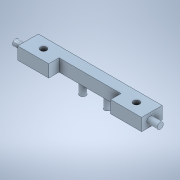
# Autodesk Inventor part: Fuehrungslagerhalter_v1
Saved by Autodesk Inventor 2022 (Build 260153000, 153)
## iProperties
Created: 2022-04-21
Part Number: Fuehrungslagerhalter_v1
Material: Generisch
Document SubType Name: Modeling
Designer: 123St
Density: 1 g/cm^3
Appearance: Stahlblau
Author: 123St
Autodesk Inventor part; units mm, degrees
ref_plane "YZ Plane" through (0, 0, 0) normal (1, 0, 0) x (0, 1, 0)
ref_plane "XZ Plane" through (0, 0, 0) normal (0, 1, 0) x (-1, 0, 0)
ref_plane "XY Plane" through (0, 0, 0) normal (0, 0, 1) x (1, 0, 0)
sketch "Skizze1" plane through (0, 0, 0) normal (0, 1, 0) x (-1, 0, 0)
  line L0 (30, 0.2989) -> (30, 10.2989)
  line L1 (30, 10.2989) -> (15, 10.2989)
  line L2 (15, 10.2989) -> (15, 5.2989)
  line L3 (15, 5.2989) -> (-15, 5.2989)
  line L4 (-15, 5.2989) -> (-15, 10.2989)
  line L5 (-15, 10.2989) -> (-30, 10.2989)
  line L6 (-30, 10.2989) -> (-30, 0.2989)
  line L7 (-30, 0.2989) -> (30, 0.2989)
  line L8 (0, -2.0598) -> (0, 12.3587) projected
  point P0 (0, 0)
  dimension "d0" = 30
  dimension "d1" = 5
  dimension "d2" = 15
  dimension "d3" = 15
  dimension "d4" = 15
  dimension "d5" = 5
  constraints: 16 end point, 6 perpendicular, 2 point on line, 1 vertical
  measures "d0" distance of L2.end L3.end
  measures "d1" distance of L1.end L2.end
  measures "d2" distance between parallel lines of L8 L4
  measures "d3" distance of L0.end L1.end
  measures "d4" distance of L4.end L5.end
  measures "d5" distance between parallel lines of L3 L7
extrude "Extrusion1" add sketch "Skizze1" along normal blind 6
sketch "Skizze2" plane through (30, 0, 10.2989) normal (1, 0, 0) x (0, 0, -1)
  circle A0 centre (4, 3) radius 1.5
  line L0 (0, 0) -> (0, 6) projected
  line L1 (0, 6) -> (10, 6) projected
  point P0 (10.2989, 0)
  dimension "d8" = 3
  dimension "d9" = 4
  dimension "d10" = 3
  constraints: 1 centre point
  measures "d8" diameter of A0
  measures "d9" distance from line of L0 A0.centre
  measures "d10" distance from line of L1 A0.centre
extrude "Extrusion2" add sketch "Skizze2" along normal blind 5
sketch "Skizze4" plane through (-30, 0, 0.2989) normal (-1, 0, 0) x (0, 0, 1)
  circle A0 centre (6, 3) radius 1.5 projected
  circle A1 centre (6, 3) radius 1.5
  line L0 (10, 0) -> (10, 6) projected
  line L1 (0, 0) -> (10, 0) projected
  point P0 (-0.2989, 0)
  dimension "d21" = 4
  dimension "d22" = 3
  constraints: 1 centre point, 1 coincident
  measures "d21" distance from line of L0 A1.centre
  measures "d22" distance from line of L1 A1.centre
extrude "Extrusion4" add sketch "Skizze4" along normal blind 5
sketch "Skizze5" plane through (0, 6, 0) normal (0, 1, 0) x (1, 0, 0)
  circle A0 centre (-22.5, -5.2989) radius 1.5
  circle A1 centre (22.5, -5.2989) radius 1.5
  line L0 (-30, -10.2989) -> (-15, -10.2989) projected
  line L1 (-30, -0.2989) -> (-30, -10.2989) projected
  line L2 (30, -10.2989) -> (30, -0.2989) projected
  line L3 (15, -10.2989) -> (30, -10.2989) projected
  point P0 (0, 0)
  dimension "d25" = 5
  dimension "d26" = 7.5
  dimension "d27" = 7.5
  dimension "d28" = 5
  dimension "d29" = 3
  dimension "d30" = 3
  constraints: 2 centre point
  measures "d25" distance from line of L0 A0.centre
  measures "d26" distance from line of L1 A0.centre
  measures "d27" distance from line of L2 A1.centre
  measures "d28" distance from line of L3 A1.centre
  measures "d29" diameter of A0
  measures "d30" diameter of A1
extrude "Extrusion5" cut sketch "Skizze5" against normal blind 6
sketch "Skizze6" plane through (0, 0, 0) normal (0, -1, 0) x (1, 0, 0)
  circle A0 centre (-6, 2.7989) radius 1.5
  circle A1 centre (6, 2.7989) radius 1.5
  line L0 (-30, 0.2989) -> (-30, 10.2989) projected
  line L1 (-30, 10.2989) -> (-15, 10.2989) projected
  line L2 (15, 10.2989) -> (30, 10.2989) projected
  line L3 (30, 10.2989) -> (30, 0.2989) projected
  point P0 (0, 0)
  dimension "d33" = 3
  dimension "d34" = 3
  dimension "d36" = 7.5
  dimension "d37" = 7.5
  dimension "d41" = 6
  dimension "d42" = 6
  constraints: 2 centre point
  measures "d33" diameter of A1
  measures "d34" diameter of A0
  measures "d36" distance from line of L1 A0.centre
  measures "d37" distance from line of L2 A1.centre
  measures "d41" horizontal distance of point (0, 0) A0.centre
  measures "d42" horizontal distance of point (0, 0) A1.centre
extrude "Extrusion6" add sketch "Skizze6" along normal blind 6
equation "\"d2\" = 0.5 * d0"
